Autodesk Inventor part; units mm, degrees
(part 2 of 3)
  arc A507 (33.3756, 32.7365) -> (33.2415, 32.8706) centre (33.2415, 32.7365) ccw
  arc A508 (33.3439, 32.7365) -> (33.4073, 32.7365) centre (33.3756, 32.7365) ccw
  arc A509 (33.2415, 32.9023) -> (33.2415, 32.8388) centre (33.2415, 32.8705) ccw
  line L202 (33.3756, 32.7365) -> (33.3756, 32.6025)
  arc A510 (33.3438, 32.6025) -> (33.4074, 32.6025) centre (33.3756, 32.6025) ccw
  arc A511 (33.4074, 32.7365) -> (33.3438, 32.7365) centre (33.3756, 32.7365) ccw
  arc A512 (33.0137, 33.4375) -> (32.893, 33.3169) centre (33.0137, 33.3168) ccw
  arc A513 (33.0137, 33.4058) -> (33.0137, 33.4693) centre (33.0137, 33.4376) ccw
  arc A514 (32.8612, 33.3169) -> (32.9247, 33.3169) centre (32.8929, 33.3169) ccw
  arc A515 (32.893, 33.3169) -> (33.0002, 33.1694) centre (33.048, 33.3168) ccw
  arc A516 (32.9247, 33.3169) -> (32.8613, 33.3169) centre (32.893, 33.3169) ccw
  arc A517 (32.9905, 33.1392) -> (33.01, 33.1996) centre (33.0002, 33.1694) ccw
  arc A518 (33.1075, 33.3973) -> (33.0137, 33.4375) centre (33.0137, 33.308) ccw
  arc A519 (33.0137, 33.4693) -> (33.0137, 33.4058) centre (33.0137, 33.4376) ccw
  line L203 (33.1075, 33.3973) -> (33.3756, 33.1694)
  arc A520 (33.355, 33.1452) -> (33.3962, 33.1936) centre (33.3756, 33.1694) ccw
  arc A521 (33.1281, 33.4215) -> (33.0869, 33.3731) centre (33.1075, 33.3973) ccw
  line L204 (33.3756, 33.1694) -> (33.3756, 33.4375)
  arc A522 (33.4074, 33.4375) -> (33.3438, 33.4375) centre (33.3756, 33.4375) ccw
  arc A523 (33.3438, 33.1694) -> (33.4074, 33.1694) centre (33.3756, 33.1694) ccw
  arc A524 (27.3812, 21.5392) -> (27.3304, 21.5392) centre (27.3558, 21.5392) ccw
  arc A525 (27.3304, 20.6502) -> (27.3812, 20.6502) centre (27.3558, 20.6502) ccw
  line L205 (27.3558, 21.5392) -> (27.6027, 21.5392)
  arc A526 (27.6027, 21.5138) -> (27.6027, 21.5646) centre (27.6027, 21.5392) ccw
  arc A527 (27.3558, 21.5646) -> (27.3558, 21.5138) centre (27.3558, 21.5392) ccw
  arc A528 (27.6027, 21.0453) -> (27.6027, 21.5392) centre (27.6027, 21.2923) ccw
  arc A529 (27.6027, 21.0707) -> (27.6027, 21.0199) centre (27.6027, 21.0453) ccw
  arc A530 (27.6027, 21.5646) -> (27.6027, 21.5138) centre (27.6027, 21.5392) ccw
  line L206 (27.6027, 21.0453) -> (27.3558, 21.0453)
  arc A531 (27.6027, 21.0199) -> (27.6027, 21.0707) centre (27.6027, 21.0453) ccw
  line L207 (27.8497, 20.6502) -> (27.6521, 21.0453)
  arc A532 (27.6748, 21.0567) -> (27.6294, 21.034) centre (27.6521, 21.0453) ccw
  arc A533 (27.827, 20.6388) -> (27.8724, 20.6616) centre (27.8497, 20.6502) ccw
  arc A534 (28.7347, 21.317) -> (28.5124, 21.5392) centre (28.5124, 21.3169) ccw
  arc A535 (28.7093, 21.317) -> (28.7601, 21.317) centre (28.7347, 21.317) ccw
  arc A536 (28.5124, 21.5646) -> (28.5124, 21.5138) centre (28.5124, 21.5392) ccw
  arc A537 (33.0845, 33.3754) -> (33.1305, 33.4192) centre (33.1075, 33.3973) ccw
  line L208 (23.8252, 31.5903) -> (22.9362, 31.5903)
  arc A538 (22.9362, 31.6157) -> (22.9362, 31.5649) centre (22.9362, 31.5903) ccw
  arc A539 (23.8252, 31.5649) -> (23.8252, 31.6157) centre (23.8252, 31.5903) ccw
  line L209 (22.9362, 31.5903) -> (22.9362, 31.8373)
  arc A540 (22.9616, 31.8373) -> (22.9108, 31.8373) centre (22.9362, 31.8373) ccw
  arc A541 (22.9108, 31.5903) -> (22.9616, 31.5903) centre (22.9362, 31.5903) ccw
  arc A542 (23.4301, 31.8373) -> (22.9362, 31.8373) centre (23.1831, 31.8373) ccw
  arc A543 (23.4047, 31.8373) -> (23.4555, 31.8373) centre (23.4301, 31.8373) ccw
  arc A544 (22.9108, 31.8373) -> (22.9616, 31.8373) centre (22.9362, 31.8373) ccw
  line L210 (23.4301, 31.8373) -> (23.4301, 31.5903)
  arc A545 (23.4047, 31.5903) -> (23.4555, 31.5903) centre (23.4301, 31.5903) ccw
  arc A546 (23.4555, 31.8373) -> (23.4047, 31.8373) centre (23.4301, 31.8373) ccw
  line L211 (23.8252, 32.0842) -> (23.4301, 31.8867)
  arc A547 (23.4187, 31.9094) -> (23.4414, 31.8639) centre (23.4301, 31.8867) ccw
  arc A548 (23.8366, 32.0615) -> (23.8138, 32.1069) centre (23.8252, 32.0842) ccw
  line L212 (22.9362, 32.6729) -> (23.6276, 32.4753)
  arc A549 (23.6207, 32.4509) -> (23.6346, 32.4997) centre (23.6276, 32.4753) ccw
  arc A550 (28.5124, 21.5392) -> (28.2408, 21.3416) centre (28.5124, 21.2537) ccw
  arc A551 (22.9432, 32.6973) -> (22.9292, 32.6484) centre (22.9362, 32.6728) ccw
  line L213 (23.6276, 32.4753) -> (23.6276, 32.9692)
  arc A552 (23.653, 32.9692) -> (23.6022, 32.9692) centre (23.6276, 32.9692) ccw
  arc A553 (23.6022, 32.4753) -> (23.653, 32.4753) centre (23.6276, 32.4753) ccw
  line L214 (23.4301, 32.821) -> (23.8252, 32.821)
  arc A554 (23.8252, 32.7956) -> (23.8252, 32.8464) centre (23.8252, 32.821) ccw
  arc A555 (23.4301, 32.8464) -> (23.4301, 32.7956) centre (23.4301, 32.821) ccw
  arc A556 (29.2213, 23.5458) -> (29.2721, 23.5458) centre (29.2467, 23.5458) ccw
  arc A557 (29.2721, 23.7927) -> (29.2213, 23.7927) centre (29.2467, 23.7927) ccw
  line L215 (29.6418, 24.0397) -> (29.2467, 23.8421)
  arc A558 (29.2353, 23.8648) -> (29.258, 23.8194) centre (29.2467, 23.8421) ccw
  arc A559 (29.6532, 24.017) -> (29.6304, 24.0624) centre (29.6418, 24.0397) ccw
  line L216 (29.6418, 24.4308) -> (29.6418, 24.6777)
  arc A560 (29.6672, 24.6777) -> (29.6164, 24.6777) centre (29.6418, 24.6777) ccw
  arc A561 (29.6164, 24.4308) -> (29.6672, 24.4308) centre (29.6418, 24.4308) ccw
  arc A562 (29.6418, 24.6777) -> (29.1479, 24.6777) centre (29.3948, 24.6777) ccw
  arc A563 (29.6164, 24.6777) -> (29.6672, 24.6777) centre (29.6418, 24.6777) ccw
  arc A564 (29.1225, 24.6777) -> (29.1733, 24.6777) centre (29.1479, 24.6777) ccw
  line L217 (28.7528, 24.4308) -> (28.7528, 24.7271)
  arc A565 (28.7782, 24.7271) -> (28.7274, 24.7271) centre (28.7528, 24.7271) ccw
  arc A566 (28.7274, 24.4308) -> (28.7782, 24.4308) centre (28.7528, 24.4308) ccw
  arc A567 (29.1479, 24.7271) -> (28.7528, 24.7271) centre (28.9504, 24.7271) ccw
  arc A568 (29.1225, 24.7271) -> (29.1733, 24.7271) centre (29.1479, 24.7271) ccw
  arc A569 (28.7274, 24.7271) -> (28.7782, 24.7271) centre (28.7528, 24.7271) ccw
  line L218 (29.1479, 24.7271) -> (29.1479, 24.5296)
  arc A570 (29.1225, 24.5296) -> (29.1733, 24.5296) centre (29.1479, 24.5296) ccw
  arc A571 (29.1733, 24.7271) -> (29.1225, 24.7271) centre (29.1479, 24.7271) ccw
  arc A572 (31.2023, 14.7715) -> (31.2023, 14.8223) centre (31.2023, 14.7969) ccw
  arc A573 (28.5124, 21.5138) -> (28.5124, 21.5646) centre (28.5124, 21.5392) ccw
  arc A574 (28.2166, 21.3495) -> (28.2649, 21.3338) centre (28.2408, 21.3417) ccw
  line L219 (31.4492, 14.4018) -> (31.2517, 14.7969)
  arc A575 (28.6606, 21.1441) -> (28.7347, 21.317) centre (28.496, 21.317) ccw
  arc A576 (28.6431, 21.1625) -> (28.6781, 21.1257) centre (28.6606, 21.1441) ccw
  arc A577 (28.7601, 21.3169) -> (28.7093, 21.317) centre (28.7347, 21.317) ccw
  line L220 (28.6606, 21.1441) -> (28.2408, 20.6502)
  line L221 (29.6418, 23.5458) -> (28.7528, 23.5458)
  arc A578 (28.7528, 23.5712) -> (28.7528, 23.5204) centre (28.7528, 23.5458) ccw
  arc A579 (29.6418, 23.5204) -> (29.6418, 23.5712) centre (29.6418, 23.5458) ccw
  line L222 (28.7528, 23.5458) -> (28.7528, 23.7927)
  arc A580 (28.7782, 23.7927) -> (28.7274, 23.7927) centre (28.7528, 23.7927) ccw
  arc A581 (28.7274, 23.5458) -> (28.7782, 23.5458) centre (28.7528, 23.5458) ccw
  arc A582 (29.2467, 23.7927) -> (28.7528, 23.7927) centre (28.9997, 23.7927) ccw
  arc A583 (29.2213, 23.7927) -> (29.2721, 23.7927) centre (29.2467, 23.7927) ccw
  arc A584 (28.2214, 20.6667) -> (28.2601, 20.6337) centre (28.2408, 20.6502) ccw
  arc A585 (28.6799, 21.1276) -> (28.6412, 21.1605) centre (28.6606, 21.1441) ccw
  line L223 (28.2408, 20.6502) -> (28.7347, 20.6502)
  arc A586 (28.7347, 20.6248) -> (28.7347, 20.6756) centre (28.7347, 20.6502) ccw
  arc A587 (28.2408, 20.6756) -> (28.2408, 20.6248) centre (28.2408, 20.6502) ccw
  arc A588 (31.2744, 14.8083) -> (31.2289, 14.7856) centre (31.2516, 14.7969) ccw
  arc A589 (30.9553, 14.8223) -> (30.9553, 14.7715) centre (30.9553, 14.7969) ccw
  line L224 (31.2023, 14.7969) -> (30.9553, 14.7969)
  arc A590 (31.2023, 15.3162) -> (31.2023, 15.2654) centre (31.2023, 15.2908) ccw
  arc A591 (31.2023, 14.8223) -> (31.2023, 14.7715) centre (31.2023, 14.7969) ccw
  arc A592 (31.2023, 14.7969) -> (31.2023, 15.2908) centre (31.2023, 15.0439) ccw
  arc A593 (30.9553, 15.3162) -> (30.9553, 15.2654) centre (30.9553, 15.2908) ccw
  arc A594 (31.2023, 15.2654) -> (31.2023, 15.3162) centre (31.2023, 15.2908) ccw
  line L225 (30.9553, 15.2908) -> (31.2023, 15.2908)
  arc A595 (30.9299, 14.4018) -> (30.9807, 14.4018) centre (30.9553, 14.4018) ccw
  arc A596 (30.9807, 15.2908) -> (30.9299, 15.2908) centre (30.9553, 15.2908) ccw
  line L226 (30.9553, 14.4018) -> (30.9553, 15.2908)
  arc A597 (31.4265, 14.3904) -> (31.4719, 14.4132) centre (31.4492, 14.4018) ccw
  arc A598 (41.6076, 4.6462) -> (41.6076, 4.5954) centre (41.6076, 4.6208) ccw
  arc A599 (42.2567, 4.5954) -> (42.2567, 4.6462) centre (42.2567, 4.6208) ccw
  line L227 (41.6076, 4.6208) -> (42.2567, 4.6208)
  arc A600 (42.1787, 5.2535) -> (42.14, 5.2864) centre (42.1594, 5.2699) ccw
  arc A601 (41.5883, 4.6373) -> (41.627, 4.6043) centre (41.6077, 4.6208) ccw
  line L228 (42.1594, 5.2699) -> (41.6076, 4.6208)
  arc A602 (42.2821, 5.4971) -> (42.2313, 5.4971) centre (42.2567, 5.4971) ccw
  arc A603 (42.1418, 5.2883) -> (42.1769, 5.2515) centre (42.1594, 5.2699) ccw
  arc A604 (42.1594, 5.2699) -> (42.2567, 5.4971) centre (41.943, 5.497) ccw
  arc A605 (41.5834, 5.5374) -> (41.6318, 5.5217) centre (41.6076, 5.5296) ccw
  arc A606 (41.9646, 5.7638) -> (41.9646, 5.8146) centre (41.9646, 5.7892) ccw
  arc A607 (41.9646, 5.7892) -> (41.6076, 5.5296) centre (41.9646, 5.414) ccw
  arc A608 (41.9646, 5.8146) -> (41.9646, 5.7638) centre (41.9646, 5.7892) ccw
  arc A609 (42.2313, 5.4971) -> (42.2821, 5.4971) centre (42.2567, 5.4971) ccw
  arc A610 (42.2567, 5.4971) -> (41.9646, 5.7892) centre (41.9646, 5.4971) ccw
  arc A611 (40.8206, 4.5954) -> (40.8206, 4.6462) centre (40.8206, 4.6208) ccw
  arc A612 (40.6908, 4.6462) -> (40.6908, 4.5954) centre (40.6908, 4.6208) ccw
  line L229 (40.8206, 4.6208) -> (40.6908, 4.6208)
  arc A613 (41.1057, 4.8804) -> (41.0549, 4.8804) centre (41.0803, 4.8804) ccw
  arc A614 (40.8206, 4.6462) -> (40.8206, 4.5954) centre (40.8206, 4.6208) ccw
  arc A615 (40.8206, 4.6208) -> (41.0803, 4.8804) centre (40.8206, 4.8805) ccw
  arc A616 (41.1057, 5.7892) -> (41.0549, 5.7892) centre (41.0803, 5.7892) ccw
  arc A617 (41.0549, 4.8804) -> (41.1057, 4.8804) centre (41.0803, 4.8804) ccw
  line L230 (41.0803, 5.7892) -> (41.0803, 4.8804)
  arc A618 (28.2702, 18.8976) -> (28.2702, 18.8468) centre (28.2702, 18.8722) ccw
  arc A619 (28.7641, 18.8468) -> (28.7641, 18.8976) centre (28.7641, 18.8722) ccw
  line L231 (28.2702, 18.8722) -> (28.7641, 18.8722)
  arc A620 (28.5425, 19.7612) -> (28.4917, 19.7612) centre (28.5171, 19.7612) ccw
  arc A621 (28.4917, 18.8722) -> (28.5425, 18.8722) centre (28.5171, 18.8722) ccw
  line L232 (28.5171, 19.7612) -> (28.5171, 18.8722)
  arc A622 (28.2543, 19.5835) -> (28.2861, 19.5438) centre (28.2702, 19.5637) ccw
  arc A623 (28.533, 19.7414) -> (28.5013, 19.781) centre (28.5172, 19.7612) ccw
  line L233 (28.2702, 19.5636) -> (28.5171, 19.7612)
  arc A624 (29.5815, 18.9957) -> (29.6556, 19.3167) centre (28.9231, 19.3167) ccw
  arc A625 (31.3975, 16.1676) -> (31.4421, 16.192) centre (31.4198, 16.1798) ccw
  arc A626 (31.1458, 16.7352) -> (31.1012, 16.7109) centre (31.1235, 16.7231) ccw
  line L234 (31.4198, 16.1798) -> (31.1235, 16.7231)
  arc A627 (31.4386, 17.0517) -> (31.401, 17.0859) centre (31.4198, 17.0688) ccw
  arc A628 (30.9071, 16.5426) -> (30.9447, 16.5084) centre (30.9259, 16.5255) ccw
  line L235 (31.4198, 17.0688) -> (30.9259, 16.5255)
  arc A629 (30.9005, 16.1798) -> (30.9513, 16.1798) centre (30.9259, 16.1798) ccw
  arc A630 (30.9513, 17.0688) -> (30.9005, 17.0688) centre (30.9259, 17.0688) ccw
  line L236 (30.9259, 16.1798) -> (30.9259, 17.0688)
  arc A631 (30.0191, 16.3932) -> (30.0588, 16.3615) centre (30.0389, 16.3773) ccw
  arc A632 (30.4539, 16.8554) -> (30.4143, 16.8871) centre (30.4341, 16.8712) ccw
  line L237 (30.039, 16.3774) -> (30.4341, 16.8712)
  arc A633 (30.4334, 16.295) -> (30.3854, 16.3115) centre (30.4094, 16.3032) ccw
  arc A634 (30.2365, 16.2052) -> (30.2365, 16.1544) centre (30.2365, 16.1798) ccw
  arc A635 (30.2365, 16.1798) -> (30.4094, 16.3033) centre (30.2365, 16.3626) ccw
  arc A636 (30.5089, 16.6243) -> (30.4581, 16.6243) centre (30.4835, 16.6243) ccw
  arc A637 (30.3866, 16.3144) -> (30.4322, 16.2921) centre (30.4094, 16.3032) ccw
  arc A638 (30.4094, 16.3033) -> (30.4835, 16.6243) centre (29.751, 16.6243) ccw
  arc A639 (30.2365, 16.1544) -> (30.2365, 16.2052) centre (30.2365, 16.1798) ccw
  arc A640 (30.0877, 16.3115) -> (30.0396, 16.295) centre (30.0637, 16.3032) ccw
  arc A641 (30.0637, 16.3033) -> (30.2365, 16.1798) centre (30.2365, 16.3625) ccw
  arc A642 (30.0408, 16.2921) -> (30.0865, 16.3144) centre (30.0637, 16.3032) ccw
  arc A643 (30.015, 16.6243) -> (29.9642, 16.6243) centre (29.9896, 16.6243) ccw
  arc A644 (29.9896, 16.6243) -> (30.0637, 16.3033) centre (30.7221, 16.6243) ccw
  arc A645 (30.4322, 16.9565) -> (30.3866, 16.9342) centre (30.4094, 16.9453) ccw
  arc A646 (30.4581, 16.6243) -> (30.5089, 16.6243) centre (30.4835, 16.6243) ccw
  arc A647 (30.4835, 16.6243) -> (30.4094, 16.9453) centre (29.751, 16.6243) ccw
  arc A648 (30.2365, 17.0942) -> (30.2365, 17.0434) centre (30.2365, 17.0688) ccw
  arc A649 (30.3854, 16.9371) -> (30.4334, 16.9536) centre (30.4094, 16.9454) ccw
  arc A650 (30.0396, 16.9536) -> (30.0877, 16.9371) centre (30.0637, 16.9454) ccw
  arc A651 (30.2365, 17.0434) -> (30.2365, 17.0942) centre (30.2365, 17.0688) ccw
  arc A652 (30.2365, 17.0688) -> (30.0637, 16.9453) centre (30.2365, 16.8861) ccw
  arc A653 (29.9642, 16.6243) -> (30.015, 16.6243) centre (29.9896, 16.6243) ccw
  arc A654 (30.0865, 16.9342) -> (30.0408, 16.9565) centre (30.0637, 16.9453) ccw
  arc A655 (30.0637, 16.9453) -> (29.9896, 16.6243) centre (30.7221, 16.6243) ccw
  arc A656 (29.0981, 16.2052) -> (29.0981, 16.1544) centre (29.0981, 16.1798) ccw
  arc A657 (29.5919, 16.1544) -> (29.5919, 16.2052) centre (29.5919, 16.1798) ccw
  line L238 (29.0981, 16.1798) -> (29.5919, 16.1798)
  arc A658 (29.3704, 17.0688) -> (29.3196, 17.0688) centre (29.345, 17.0688) ccw
  arc A659 (29.3196, 16.1798) -> (29.3704, 16.1798) centre (29.345, 16.1798) ccw
  line L239 (29.345, 17.0688) -> (29.345, 16.1798)
  arc A660 (29.0822, 16.8911) -> (29.1139, 16.8514) centre (29.0981, 16.8713) ccw
  arc A661 (29.3609, 17.049) -> (29.3291, 17.0886) centre (29.345, 17.0688) ccw
  line L240 (29.0981, 16.8712) -> (29.345, 17.0688)
  arc A662 (30.5697, 18.86) -> (30.6142, 18.8844) centre (30.592, 18.8722) ccw
  arc A663 (30.3179, 19.4276) -> (30.2733, 19.4033) centre (30.2956, 19.4154) ccw
  line L241 (30.592, 18.8722) -> (30.2956, 19.4155)
  arc A664 (30.6107, 19.7441) -> (30.5732, 19.7783) centre (30.592, 19.7612) ccw
  arc A665 (30.0793, 19.235) -> (30.1169, 19.2008) centre (30.0981, 19.2179) ccw
  line L242 (30.592, 19.7612) -> (30.0981, 19.2179)
  arc A666 (30.0727, 18.8722) -> (30.1235, 18.8722) centre (30.0981, 18.8722) ccw
  arc A667 (30.1235, 19.7612) -> (30.0727, 19.7612) centre (30.0981, 19.7612) ccw
  line L243 (30.0981, 18.8722) -> (30.0981, 19.7612)
  arc A668 (29.1913, 19.0856) -> (29.231, 19.0539) centre (29.2112, 19.0697) ccw
  arc A669 (29.6261, 19.5478) -> (29.5864, 19.5795) centre (29.6063, 19.5636) ccw
  line L244 (29.2111, 19.0698) -> (29.6062, 19.5636)
  arc A670 (29.6056, 18.9874) -> (29.5575, 19.0039) centre (29.5816, 18.9957) ccw
  arc A671 (29.4087, 18.8976) -> (29.4087, 18.8468) centre (29.4087, 18.8722) ccw
  arc A672 (29.4087, 18.8722) -> (29.5815, 18.9957) centre (29.4087, 19.0549) ccw
  arc A673 (29.681, 19.3167) -> (29.6302, 19.3167) centre (29.6556, 19.3167) ccw
  arc A674 (29.5587, 19.0068) -> (29.6044, 18.9845) centre (29.5816, 18.9956) ccw
  arc A675 (30.4094, 16.9453) -> (30.2365, 17.0688) centre (30.2365, 16.886) ccw
  arc A676 (29.4087, 18.8468) -> (29.4087, 18.8976) centre (29.4087, 18.8722) ccw
  arc A677 (29.2598, 19.0039) -> (29.2118, 18.9874) centre (29.2358, 18.9957) ccw
  arc A678 (29.2358, 18.9957) -> (29.4087, 18.8722) centre (29.4087, 19.055) ccw
  arc A679 (29.213, 18.9845) -> (29.2587, 19.0068) centre (29.2358, 18.9956) ccw
  arc A680 (29.1871, 19.3167) -> (29.1363, 19.3167) centre (29.1617, 19.3167) ccw
  arc A681 (29.1617, 19.3167) -> (29.2358, 18.9957) centre (29.8942, 19.3167) ccw
  arc A682 (29.6044, 19.6489) -> (29.5587, 19.6266) centre (29.5816, 19.6378) ccw
  arc A683 (29.6302, 19.3167) -> (29.681, 19.3167) centre (29.6556, 19.3167) ccw
  arc A684 (29.6556, 19.3167) -> (29.5815, 19.6377) centre (28.9231, 19.3167) ccw
  arc A685 (29.4087, 19.7866) -> (29.4087, 19.7358) centre (29.4087, 19.7612) ccw
  arc A686 (29.5575, 19.6295) -> (29.6056, 19.646) centre (29.5816, 19.6378) ccw
  arc A687 (29.5815, 19.6377) -> (29.4087, 19.7612) centre (29.4087, 19.5785) ccw
  arc A688 (29.2118, 19.646) -> (29.2598, 19.6295) centre (29.2358, 19.6378) ccw
  arc A689 (29.4087, 19.7358) -> (29.4087, 19.7866) centre (29.4087, 19.7612) ccw
  arc A690 (29.4087, 19.7612) -> (29.2358, 19.6377) centre (29.4087, 19.5784) ccw
  arc A691 (29.1363, 19.3167) -> (29.1871, 19.3167) centre (29.1617, 19.3167) ccw
  arc A692 (29.2587, 19.6266) -> (29.213, 19.6489) centre (29.2358, 19.6378) ccw
  arc A693 (29.2358, 19.6377) -> (29.1617, 19.3167) centre (29.8942, 19.3167) ccw
  arc A694 (21.463, 33.401) -> (21.717, 33.401) centre (21.59, 33.401) ccw
  line L245 (21.59, 34.29) -> (21.59, 33.401)
  arc A695 (34.671, 33.02) -> (36.83, 30.861) centre (36.83, 33.02) ccw
  arc A696 (35.179, 33.02) -> (36.83, 31.369) centre (36.83, 33.02) ccw
  arc A697 (37.973, 33.02) -> (36.83, 34.163) centre (36.83, 33.02) ccw
  arc A698 (35.687, 33.02) -> (36.83, 31.877) centre (36.83, 33.02) ccw
  arc A699 (24.765, 30.5308) -> (24.765, 30.4292) centre (24.765, 30.48) ccw
  arc A700 (28.575, 30.4292) -> (28.575, 30.5308) centre (28.575, 30.48) ccw
  line L246 (24.765, 30.48) -> (28.575, 30.48)
  arc A701 (24.511, 33.02) -> (26.67, 30.861) centre (26.67, 33.02) ccw
  arc A702 (28.829, 33.02) -> (26.67, 35.179) centre (26.67, 33.02) ccw
  arc A703 (25.019, 33.02) -> (26.67, 31.369) centre (26.67, 33.02) ccw
  arc A704 (28.321, 33.02) -> (26.67, 34.671) centre (26.67, 33.02) ccw
  arc A705 (25.527, 33.02) -> (26.67, 31.877) centre (26.67, 33.02) ccw
  arc A706 (27.813, 33.02) -> (26.67, 34.163) centre (26.67, 33.02) ccw
  arc A707 (21.463, 26.67) -> (21.717, 26.67) centre (21.59, 26.67) ccw
  arc A708 (21.717, 27.559) -> (21.463, 27.559) centre (21.59, 27.559) ccw
  line L247 (21.59, 26.67) -> (21.59, 27.559)
  arc A709 (30.861, 22.225) -> (31.115, 22.225) centre (30.988, 22.225) ccw
  line L248 (32.7604, 10.8692) -> (32.7604, 9.7008)
  arc A710 (32.4199, 10.6294) -> (32.4517, 10.5897) centre (32.4358, 10.6096) ccw
  arc A711 (32.7762, 10.8494) -> (32.7445, 10.889) centre (32.7604, 10.8692) ccw
  line L249 (32.4358, 10.6096) -> (32.7604, 10.8692)
  arc A712 (24.3483, -0.92) -> (24.4118, -0.92) centre (24.3801, -0.92) ccw
  arc A713 (24.4118, 12.08) -> (24.3483, 12.08) centre (24.3801, 12.08) ccw
  line L250 (24.38, -0.92) -> (24.38, 12.08)
  arc A714 (33.655, 16.51) -> (33.655, 16.764) centre (33.655, 16.637) ccw
  arc A715 (32.766, 16.764) -> (32.766, 16.51) centre (32.766, 16.637) ccw
  line L251 (33.655, 16.637) -> (32.766, 16.637)
  arc A716 (26.035, 16.764) -> (26.035, 16.51) centre (26.035, 16.637) ccw
  arc A717 (26.924, 16.51) -> (26.924, 16.764) centre (26.924, 16.637) ccw
  line L252 (26.035, 16.637) -> (26.924, 16.637)
  line L253 (30.988, 29.845) -> (30.988, 28.956)
  arc A718 (38.481, 33.02) -> (36.83, 34.671) centre (36.83, 33.02) ccw
  arc A719 (27.8751, 8.1788) -> (27.8751, 8.2296) centre (27.8751, 8.2042) ccw
  arc A720 (27.8751, 8.2042) -> (27.3558, 7.6849) centre (27.8751, 7.6849) ccw
  arc A721 (27.3304, 7.3604) -> (27.3812, 7.3604) centre (27.3558, 7.3604) ccw
  arc A722 (27.3812, 7.6849) -> (27.3304, 7.6849) centre (27.3558, 7.6849) ccw
  line L254 (27.3558, 7.3604) -> (27.3558, 7.6849)
  arc A723 (28.0303, 7.3604) -> (27.9795, 7.3604) centre (28.0049, 7.3604) ccw
  arc A724 (27.3812, 7.3604) -> (27.3304, 7.3604) centre (27.3558, 7.3604) ccw
  arc A725 (27.3558, 7.3604) -> (28.0049, 7.3604) centre (27.6803, 7.3604) ccw
  arc A726 (28.0303, 7.4253) -> (27.9795, 7.4253) centre (28.0049, 7.4253) ccw
  arc A727 (27.9795, 7.3604) -> (28.0303, 7.3604) centre (28.0049, 7.3604) ccw
  line L255 (28.0049, 7.4253) -> (28.0049, 7.3604)
  arc A728 (27.7453, 7.7103) -> (27.7453, 7.6595) centre (27.7453, 7.6849) ccw
  arc A729 (27.9795, 7.4253) -> (28.0303, 7.4253) centre (28.0049, 7.4253) ccw
  arc A730 (28.0049, 7.4253) -> (27.7453, 7.6849) centre (27.7453, 7.4253) ccw
  arc A731 (27.3558, 7.7103) -> (27.3558, 7.6595) centre (27.3558, 7.6849) ccw
  arc A732 (27.7453, 7.6595) -> (27.7453, 7.7103) centre (27.7453, 7.6849) ccw
  line L256 (27.3558, 7.6849) -> (27.7453, 7.6849)
  arc A733 (36.58, -0.9518) -> (36.58, -0.8882) centre (36.58, -0.92) ccw
  arc A734 (24.38, -0.8882) -> (24.38, -0.9518) centre (24.38, -0.92) ccw
  line L257 (36.58, -0.92) -> (24.38, -0.92)
  arc A735 (36.6118, 12.08) -> (36.5482, 12.08) centre (36.58, 12.08) ccw
  arc A736 (36.5482, -0.92) -> (36.6118, -0.92) centre (36.58, -0.92) ccw
  line L258 (36.58, 12.08) -> (36.58, -0.92)
  arc A737 (24.38, 12.1118) -> (24.38, 12.0482) centre (24.38, 12.08) ccw
  arc A738 (36.58, 12.0482) -> (36.58, 12.1118) centre (36.58, 12.08) ccw
  line L259 (24.38, 12.08) -> (36.58, 12.08)
  arc A739 (38.735, 35.5092) -> (38.735, 35.6108) centre (38.735, 35.56) ccw
  arc A740 (38.989, 33.02) -> (36.83, 35.179) centre (36.83, 33.02) ccw
  arc A741 (26.035, 19.431) -> (26.035, 19.177) centre (26.035, 19.304) ccw
  arc A742 (26.924, 19.177) -> (26.924, 19.431) centre (26.924, 19.304) ccw
  line L260 (26.035, 19.304) -> (26.924, 19.304)
  arc A743 (34.925, 35.6108) -> (34.925, 35.5092) centre (34.925, 35.56) ccw
  arc A744 (33.655, 19.177) -> (33.655, 19.431) centre (33.655, 19.304) ccw
  arc A745 (32.766, 19.431) -> (32.766, 19.177) centre (32.766, 19.304) ccw
  line L261 (33.655, 19.304) -> (32.766, 19.304)
  line L262 (38.735, 35.56) -> (34.925, 35.56)
  arc A746 (30.861, 28.956) -> (31.115, 28.956) centre (30.988, 28.956) ccw
  arc A747 (31.115, 29.845) -> (30.861, 29.845) centre (30.988, 29.845) ccw
  line L263 (30.988, 22.225) -> (30.988, 23.114)
  arc A748 (31.115, 23.114) -> (30.861, 23.114) centre (30.988, 23.114) ccw
  arc A749 (21.717, 34.29) -> (21.463, 34.29) centre (21.59, 34.29) ccw
  arc A750 (32.4358, 9.7262) -> (32.4358, 9.6754) centre (32.4358, 9.7008) ccw
  arc A751 (33.0849, 9.6754) -> (33.0849, 9.7262) centre (33.0849, 9.7008) ccw
  line L264 (32.4358, 9.7008) -> (33.0849, 9.7008)
  arc A752 (32.7858, 10.8692) -> (32.735, 10.8692) centre (32.7604, 10.8692) ccw
  arc A753 (32.735, 9.7008) -> (32.7858, 9.7008) centre (32.7604, 9.7008) ccw
  arc A754 (27.3304, 7.6849) -> (27.3812, 7.6849) centre (27.3558, 7.6849) ccw
  arc A755 (26.2001, 34.29) -> (27.1399, 34.29) centre (26.67, 34.29) ccw
  arc A756 (27.1399, 34.29) -> (26.2001, 34.29) centre (26.67, 34.29) ccw
  arc A757 (26.2001, 34.29) -> (27.1399, 34.29) centre (26.67, 34.29) ccw
  arc A758 (27.1399, 34.29) -> (26.2001, 34.29) centre (26.67, 34.29) ccw
  arc A759 (26.2001, 31.75) -> (27.1399, 31.75) centre (26.67, 31.75) ccw
  arc A760 (27.1399, 31.75) -> (26.2001, 31.75) centre (26.67, 31.75) ccw
  arc A761 (26.2001, 31.75) -> (27.1399, 31.75) centre (26.67, 31.75) ccw
  arc A762 (27.1399, 31.75) -> (26.2001, 31.75) centre (26.67, 31.75) ccw
  arc A763 (37.2999, 31.75) -> (36.3601, 31.75) centre (36.83, 31.75) ccw
  arc A764 (36.3601, 31.75) -> (37.2999, 31.75) centre (36.83, 31.75) ccw
  arc A765 (37.2999, 31.75) -> (36.3601, 31.75) centre (36.83, 31.75) ccw
  arc A766 (36.3601, 31.75) -> (37.2999, 31.75) centre (36.83, 31.75) ccw
  arc A767 (37.2999, 34.29) -> (36.3601, 34.29) centre (36.83, 34.29) ccw
  arc A768 (36.3601, 34.29) -> (37.2999, 34.29) centre (36.83, 34.29) ccw
  arc A769 (37.2999, 34.29) -> (36.3601, 34.29) centre (36.83, 34.29) ccw
  arc A770 (36.3601, 34.29) -> (37.2999, 34.29) centre (36.83, 34.29) ccw
  arc A771 (44.704, 11.942) -> (44.704, 12.696) centre (44.704, 12.319) ccw
  arc A772 (44.704, 12.696) -> (44.704, 11.942) centre (44.704, 12.319) ccw
  arc A773 (44.704, 11.942) -> (44.704, 12.696) centre (44.704, 12.319) ccw
  arc A774 (44.704, 12.696) -> (44.704, 11.942) centre (44.704, 12.319) ccw
  arc A775 (42.164, 11.942) -> (42.164, 12.696) centre (42.164, 12.319) ccw
  arc A776 (42.164, 12.696) -> (42.164, 11.942) centre (42.164, 12.319) ccw
  arc A777 (42.164, 11.942) -> (42.164, 12.696) centre (42.164, 12.319) ccw
  arc A778 (42.164, 12.696) -> (42.164, 11.942) centre (42.164, 12.319) ccw
  arc A779 (39.624, 11.942) -> (39.624, 12.696) centre (39.624, 12.319) ccw
  arc A780 (39.624, 12.696) -> (39.624, 11.942) centre (39.624, 12.319) ccw
  arc A781 (39.624, 11.942) -> (39.624, 12.696) centre (39.624, 12.319) ccw
  arc A782 (39.624, 12.696) -> (39.624, 11.942) centre (39.624, 12.319) ccw
  arc A783 (33.03, 9.568) -> (33.03, 10.272) centre (33.03, 9.92) ccw
  arc A784 (33.03, 10.272) -> (33.03, 9.568) centre (33.03, 9.92) ccw
  arc A785 (33.03, 9.568) -> (33.03, 10.272) centre (33.03, 9.92) ccw
  arc A786 (33.03, 10.272) -> (33.03, 9.568) centre (33.03, 9.92) ccw
  arc A787 (32.01, 7.028) -> (32.01, 7.732) centre (32.01, 7.38) ccw
  arc A788 (32.01, 7.732) -> (32.01, 7.028) centre (32.01, 7.38) ccw
  arc A789 (32.01, 7.028) -> (32.01, 7.732) centre (32.01, 7.38) ccw
  arc A790 (32.01, 7.732) -> (32.01, 7.028) centre (32.01, 7.38) ccw
  arc A791 (30.99, 9.568) -> (30.99, 10.272) centre (30.99, 9.92) ccw
  arc A792 (30.99, 10.272) -> (30.99, 9.568) centre (30.99, 9.92) ccw
  arc A793 (30.99, 9.568) -> (30.99, 10.272) centre (30.99, 9.92) ccw
  arc A794 (30.99, 10.272) -> (30.99, 9.568) centre (30.99, 9.92) ccw
  arc A795 (29.97, 7.028) -> (29.97, 7.732) centre (29.97, 7.38) ccw
  arc A796 (29.97, 7.732) -> (29.97, 7.028) centre (29.97, 7.38) ccw
  arc A797 (29.97, 7.028) -> (29.97, 7.732) centre (29.97, 7.38) ccw
  arc A798 (29.97, 7.732) -> (29.97, 7.028) centre (29.97, 7.38) ccw
  arc A799 (28.95, 9.568) -> (28.95, 10.272) centre (28.95, 9.92) ccw
  arc A800 (28.95, 10.272) -> (28.95, 9.568) centre (28.95, 9.92) ccw
  arc A801 (28.95, 9.568) -> (28.95, 10.272) centre (28.95, 9.92) ccw
  arc A802 (28.95, 10.272) -> (28.95, 9.568) centre (28.95, 9.92) ccw
  arc A803 (27.93, 7.028) -> (27.93, 7.732) centre (27.93, 7.38) ccw
  arc A804 (27.93, 7.732) -> (27.93, 7.028) centre (27.93, 7.38) ccw
  arc A805 (27.93, 7.028) -> (27.93, 7.732) centre (27.93, 7.38) ccw
  arc A806 (27.93, 7.732) -> (27.93, 7.028) centre (27.93, 7.38) ccw
  line L265 (27.6145, 17.137) -> (26.6145, 17.137)
  line L266 (26.6145, 17.137) -> (26.6145, 16.137)
  line L267 (26.6145, 16.137) -> (27.6145, 16.137)
  line L268 (27.6145, 16.137) -> (27.6145, 17.137)
  line L269 (33.0755, 17.137) -> (32.0755, 17.137)
  line L270 (32.0755, 17.137) -> (32.0755, 16.137)
  line L271 (32.0755, 16.137) -> (33.0755, 16.137)
  line L272 (33.0755, 16.137) -> (33.0755, 17.137)
  line L273 (34.1376, 16.837) -> (34.1376, 16.437)
  line L274 (34.1376, 16.437) -> (33.855, 16.1544)
  line L275 (33.855, 16.1544) -> (33.455, 16.1544)
  line L276 (33.455, 16.1544) -> (33.1724, 16.437)
  line L277 (33.1724, 16.437) -> (33.1724, 16.837)
  line L278 (33.1724, 16.837) -> (33.455, 17.1196)
  line L279 (33.455, 17.1196) -> (33.855, 17.1196)
  line L280 (33.855, 17.1196) -> (34.1376, 16.837)
  line L281 (34.1376, 16.837) -> (34.1376, 16.437)
  line L282 (34.1376, 16.837) -> (34.1376, 16.437)
  line L283 (34.1376, 16.437) -> (33.855, 16.1544)
  line L284 (33.855, 16.1544) -> (33.455, 16.1544)
  line L285 (33.455, 16.1544) -> (33.1724, 16.437)
  line L286 (33.1724, 16.437) -> (33.1724, 16.837)
  line L287 (33.1724, 16.837) -> (33.455, 17.1196)
  line L288 (33.455, 17.1196) -> (33.855, 17.1196)
  line L289 (33.855, 17.1196) -> (34.1376, 16.837)
  line L290 (34.1376, 16.837) -> (34.1376, 16.437)
  line L291 (26.5176, 16.837) -> (26.5176, 16.437)
  line L292 (26.5176, 16.437) -> (26.235, 16.1544)
  line L293 (26.235, 16.1544) -> (25.835, 16.1544)
  line L294 (25.835, 16.1544) -> (25.5524, 16.437)
  line L295 (25.5524, 16.437) -> (25.5524, 16.837)
  line L296 (25.5524, 16.837) -> (25.835, 17.1196)
  line L297 (25.835, 17.1196) -> (26.235, 17.1196)
  line L298 (26.235, 17.1196) -> (26.5176, 16.837)
  line L299 (26.5176, 16.837) -> (26.5176, 16.437)
  line L300 (26.5176, 16.837) -> (26.5176, 16.437)
  line L301 (26.5176, 16.437) -> (26.235, 16.1544)
  line L302 (26.235, 16.1544) -> (25.835, 16.1544)
  line L303 (25.835, 16.1544) -> (25.5524, 16.437)
  line L304 (25.5524, 16.437) -> (25.5524, 16.837)
  line L305 (25.5524, 16.837) -> (25.835, 17.1196)
  line L306 (25.835, 17.1196) -> (26.235, 17.1196)
  line L307 (26.235, 17.1196) -> (26.5176, 16.837)
  line L308 (26.5176, 16.837) -> (26.5176, 16.437)
  line L309 (32.0755, 18.804) -> (33.0755, 18.804)
  line L310 (33.0755, 18.804) -> (33.0755, 19.804)
  line L311 (33.0755, 19.804) -> (32.0755, 19.804)
  line L312 (32.0755, 19.804) -> (32.0755, 18.804)
  line L313 (26.6145, 18.804) -> (27.6145, 18.804)
  line L314 (27.6145, 18.804) -> (27.6145, 19.804)
  line L315 (27.6145, 19.804) -> (26.6145, 19.804)
  line L316 (26.6145, 19.804) -> (26.6145, 18.804)
  line L317 (25.5524, 19.104) -> (25.5524, 19.504)
  line L318 (25.5524, 19.504) -> (25.835, 19.7866)
  line L319 (25.835, 19.7866) -> (26.235, 19.7866)
  line L320 (26.235, 19.7866) -> (26.5176, 19.504)
  line L321 (26.5176, 19.504) -> (26.5176, 19.104)
  line L322 (26.5176, 19.104) -> (26.235, 18.8214)
  line L323 (26.235, 18.8214) -> (25.835, 18.8214)
  line L324 (25.835, 18.8214) -> (25.5524, 19.104)
  line L325 (25.5524, 19.104) -> (25.5524, 19.504)
  line L326 (25.5524, 19.104) -> (25.5524, 19.504)
  line L327 (25.5524, 19.504) -> (25.835, 19.7866)
  line L328 (25.835, 19.7866) -> (26.235, 19.7866)
  line L329 (26.235, 19.7866) -> (26.5176, 19.504)
  line L330 (26.5176, 19.504) -> (26.5176, 19.104)
  line L331 (26.5176, 19.104) -> (26.235, 18.8214)
  line L332 (26.235, 18.8214) -> (25.835, 18.8214)
  line L333 (25.835, 18.8214) -> (25.5524, 19.104)
  line L334 (25.5524, 19.104) -> (25.5524, 19.504)
  line L335 (33.1724, 19.104) -> (33.1724, 19.504)
  line L336 (33.1724, 19.504) -> (33.455, 19.7866)
  line L337 (33.455, 19.7866) -> (33.855, 19.7866)
  line L338 (33.855, 19.7866) -> (34.1376, 19.504)
  line L339 (34.1376, 19.504) -> (34.1376, 19.104)
  line L340 (34.1376, 19.104) -> (33.855, 18.8214)
  line L341 (33.855, 18.8214) -> (33.455, 18.8214)
  line L342 (33.455, 18.8214) -> (33.1724, 19.104)
  line L343 (33.1724, 19.104) -> (33.1724, 19.504)
  line L344 (33.1724, 19.104) -> (33.1724, 19.504)
  line L345 (33.1724, 19.504) -> (33.455, 19.7866)
  line L346 (33.455, 19.7866) -> (33.855, 19.7866)
  line L347 (33.855, 19.7866) -> (34.1376, 19.504)
  line L348 (34.1376, 19.504) -> (34.1376, 19.104)
  line L349 (34.1376, 19.104) -> (33.855, 18.8214)
  line L350 (33.855, 18.8214) -> (33.455, 18.8214)
  line L351 (33.455, 18.8214) -> (33.1724, 19.104)
  line L352 (33.1724, 19.104) -> (33.1724, 19.504)
  line L353 (31.488, 28.2655) -> (31.488, 29.2655)
  line L354 (31.488, 29.2655) -> (30.488, 29.2655)
  line L355 (30.488, 29.2655) -> (30.488, 28.2655)
  line L356 (30.488, 28.2655) -> (31.488, 28.2655)
  line L357 (31.488, 22.8045) -> (31.488, 23.8045)
  line L358 (31.488, 23.8045) -> (30.488, 23.8045)
  line L359 (30.488, 23.8045) -> (30.488, 22.8045)
  line L360 (30.488, 22.8045) -> (31.488, 22.8045)
  line L361 (31.188, 21.7424) -> (30.788, 21.7424)
  line L362 (30.788, 21.7424) -> (30.5054, 22.025)
  line L363 (30.5054, 22.025) -> (30.5054, 22.425)
  line L364 (30.5054, 22.425) -> (30.788, 22.7076)
  line L365 (30.788, 22.7076) -> (31.188, 22.7076)
  line L366 (31.188, 22.7076) -> (31.4706, 22.425)
  line L367 (31.4706, 22.425) -> (31.4706, 22.025)
  line L368 (31.4706, 22.025) -> (31.188, 21.7424)
  line L369 (31.188, 21.7424) -> (30.788, 21.7424)
  line L370 (31.188, 21.7424) -> (30.788, 21.7424)
  line L371 (30.788, 21.7424) -> (30.5054, 22.025)
  line L372 (30.5054, 22.025) -> (30.5054, 22.425)
  line L373 (30.5054, 22.425) -> (30.788, 22.7076)
  line L374 (30.788, 22.7076) -> (31.188, 22.7076)
  line L375 (31.188, 22.7076) -> (31.4706, 22.425)
  line L376 (31.4706, 22.425) -> (31.4706, 22.025)
  line L377 (31.4706, 22.025) -> (31.188, 21.7424)
  line L378 (31.188, 21.7424) -> (30.788, 21.7424)
  line L379 (31.188, 29.3624) -> (30.788, 29.3624)
  line L380 (30.788, 29.3624) -> (30.5054, 29.645)
  line L381 (30.5054, 29.645) -> (30.5054, 30.045)
  line L382 (30.5054, 30.045) -> (30.788, 30.3276)
  line L383 (30.788, 30.3276) -> (31.188, 30.3276)
  line L384 (31.188, 30.3276) -> (31.4706, 30.045)
  line L385 (31.4706, 30.045) -> (31.4706, 29.645)
  line L386 (31.4706, 29.645) -> (31.188, 29.3624)
  line L387 (31.188, 29.3624) -> (30.788, 29.3624)
  line L388 (31.188, 29.3624) -> (30.788, 29.3624)
  line L389 (30.788, 29.3624) -> (30.5054, 29.645)
  line L390 (30.5054, 29.645) -> (30.5054, 30.045)
  line L391 (30.5054, 30.045) -> (30.788, 30.3276)
  line L392 (30.788, 30.3276) -> (31.188, 30.3276)
  line L393 (31.188, 30.3276) -> (31.4706, 30.045)
  line L394 (31.4706, 30.045) -> (31.4706, 29.645)
  line L395 (31.4706, 29.645) -> (31.188, 29.3624)
  line L396 (31.188, 29.3624) -> (30.788, 29.3624)
  line L397 (21.09, 28.2495) -> (21.09, 27.2495)
  line L398 (21.09, 27.2495) -> (22.09, 27.2495)
  line L399 (22.09, 27.2495) -> (22.09, 28.2495)
  line L400 (22.09, 28.2495) -> (21.09, 28.2495)
  line L401 (21.09, 33.7105) -> (21.09, 32.7105)
  line L402 (21.09, 32.7105) -> (22.09, 32.7105)
  line L403 (22.09, 32.7105) -> (22.09, 33.7105)
  line L404 (22.09, 33.7105) -> (21.09, 33.7105)
  line L405 (21.39, 34.7726) -> (21.79, 34.7726)
  line L406 (21.79, 34.7726) -> (22.0726, 34.49)
  line L407 (22.0726, 34.49) -> (22.0726, 34.09)
  line L408 (22.0726, 34.09) -> (21.79, 33.8074)
  line L409 (21.79, 33.8074) -> (21.39, 33.8074)
  line L410 (21.39, 33.8074) -> (21.1074, 34.09)
  line L411 (21.1074, 34.09) -> (21.1074, 34.49)
  line L412 (21.1074, 34.49) -> (21.39, 34.7726)
  line L413 (21.39, 34.7726) -> (21.79, 34.7726)
  line L414 (21.39, 34.7726) -> (21.79, 34.7726)
  line L415 (21.79, 34.7726) -> (22.0726, 34.49)
  line L416 (22.0726, 34.49) -> (22.0726, 34.09)
  line L417 (22.0726, 34.09) -> (21.79, 33.8074)
  line L418 (21.79, 33.8074) -> (21.39, 33.8074)
  line L419 (21.39, 33.8074) -> (21.1074, 34.09)
  line L420 (21.1074, 34.09) -> (21.1074, 34.49)
  line L421 (21.1074, 34.49) -> (21.39, 34.7726)
  line L422 (21.39, 34.7726) -> (21.79, 34.7726)
  line L423 (21.39, 27.1526) -> (21.79, 27.1526)
  line L424 (21.79, 27.1526) -> (22.0726, 26.87)
  line L425 (22.0726, 26.87) -> (22.0726, 26.47)
  line L426 (22.0726, 26.47) -> (21.79, 26.1874)
  line L427 (21.79, 26.1874) -> (21.39, 26.1874)
  line L428 (21.39, 26.1874) -> (21.1074, 26.47)
  line L429 (21.1074, 26.47) -> (21.1074, 26.87)
  line L430 (21.1074, 26.87) -> (21.39, 27.1526)
  line L431 (21.39, 27.1526) -> (21.79, 27.1526)
  line L432 (21.39, 27.1526) -> (21.79, 27.1526)
  line L433 (21.79, 27.1526) -> (22.0726, 26.87)
  line L434 (22.0726, 26.87) -> (22.0726, 26.47)
  line L435 (22.0726, 26.47) -> (21.79, 26.1874)
  line L436 (21.79, 26.1874) -> (21.39, 26.1874)
  line L437 (21.39, 26.1874) -> (21.1074, 26.47)
  line L438 (21.1074, 26.47) -> (21.1074, 26.87)
  line L439 (21.1074, 26.87) -> (21.39, 27.1526)
  line L440 (21.39, 27.1526) -> (21.79, 27.1526)
  arc A807 (37.773, 16.891) -> (38.427, 16.891) centre (38.1, 16.891) ccw
  arc A808 (38.427, 16.891) -> (37.773, 16.891) centre (38.1, 16.891) ccw
  arc A809 (37.773, 16.891) -> (38.427, 16.891) centre (38.1, 16.891) ccw
  arc A810 (38.427, 16.891) -> (37.773, 16.891) centre (38.1, 16.891) ccw
  arc A811 (37.773, 19.431) -> (38.427, 19.431) centre (38.1, 19.431) ccw
  arc A812 (38.427, 19.431) -> (37.773, 19.431) centre (38.1, 19.431) ccw
  arc A813 (37.773, 19.431) -> (38.427, 19.431) centre (38.1, 19.431) ccw
  arc A814 (38.427, 19.431) -> (37.773, 19.431) centre (38.1, 19.431) ccw
  arc A815 (37.773, 21.971) -> (38.427, 21.971) centre (38.1, 21.971) ccw
  arc A816 (38.427, 21.971) -> (37.773, 21.971) centre (38.1, 21.971) ccw
  arc A817 (37.773, 21.971) -> (38.427, 21.971) centre (38.1, 21.971) ccw
  arc A818 (38.427, 21.971) -> (37.773, 21.971) centre (38.1, 21.971) ccw
  arc A819 (37.773, 24.511) -> (38.427, 24.511) centre (38.1, 24.511) ccw
  arc A820 (38.427, 24.511) -> (37.773, 24.511) centre (38.1, 24.511) ccw
  arc A821 (37.773, 24.511) -> (38.427, 24.511) centre (38.1, 24.511) ccw
  arc A822 (38.427, 24.511) -> (37.773, 24.511) centre (38.1, 24.511) ccw
  arc A823 (22.5645, 17.018) -> (21.8855, 17.018) centre (22.225, 17.018) ccw
  arc A824 (21.8855, 17.018) -> (22.5645, 17.018) centre (22.225, 17.018) ccw
  arc A825 (22.5645, 17.018) -> (21.8855, 17.018) centre (22.225, 17.018) ccw
  arc A826 (21.8855, 17.018) -> (22.5645, 17.018) centre (22.225, 17.018) ccw
  arc A827 (22.5645, 22.098) -> (21.8855, 22.098) centre (22.225, 22.098) ccw
  arc A828 (21.8855, 22.098) -> (22.5645, 22.098) centre (22.225, 22.098) ccw
  arc A829 (22.5645, 22.098) -> (21.8855, 22.098) centre (22.225, 22.098) ccw
  arc A830 (21.8855, 22.098) -> (22.5645, 22.098) centre (22.225, 22.098) ccw
  arc A831 (22.5645, 19.558) -> (21.8855, 19.558) centre (22.225, 19.558) ccw
  arc A832 (21.8855, 19.558) -> (22.5645, 19.558) centre (22.225, 19.558) ccw
  arc A833 (22.5645, 19.558) -> (21.8855, 19.558) centre (22.225, 19.558) ccw
  arc A834 (21.8855, 19.558) -> (22.5645, 19.558) centre (22.225, 19.558) ccw
  arc A835 (27.051, 12.9975) -> (27.051, 13.6725) centre (27.051, 13.335) ccw
  arc A836 (27.051, 13.6725) -> (27.051, 12.9975) centre (27.051, 13.335) ccw
  arc A837 (27.051, 12.9975) -> (27.051, 13.6725) centre (27.051, 13.335) ccw
  arc A838 (27.051, 13.6725) -> (27.051, 12.9975) centre (27.051, 13.335) ccw
  arc A839 (30.988, 12.9975) -> (30.988, 13.6725) centre (30.988, 13.335) ccw
  arc A840 (30.988, 13.6725) -> (30.988, 12.9975) centre (30.988, 13.335) ccw
  arc A841 (30.988, 12.9975) -> (30.988, 13.6725) centre (30.988, 13.335) ccw
  arc A842 (30.988, 13.6725) -> (30.988, 12.9975) centre (30.988, 13.335) ccw
  arc A843 (33.655, 26.3325) -> (33.655, 27.0075) centre (33.655, 26.67) ccw
  arc A844 (33.655, 27.0075) -> (33.655, 26.3325) centre (33.655, 26.67) ccw
  arc A845 (33.655, 26.3325) -> (33.655, 27.0075) centre (33.655, 26.67) ccw
  arc A846 (33.655, 27.0075) -> (33.655, 26.3325) centre (33.655, 26.67) ccw
  arc A847 (33.655, 22.1415) -> (33.655, 22.8165) centre (33.655, 22.479) ccw
  arc A848 (33.655, 22.8165) -> (33.655, 22.1415) centre (33.655, 22.479) ccw
  arc A849 (33.655, 22.1415) -> (33.655, 22.8165) centre (33.655, 22.479) ccw
  arc A850 (33.655, 22.8165) -> (33.655, 22.1415) centre (33.655, 22.479) ccw
  line L441 (-13.871, -1.143) -> (46.533, -1.143)
  line L442 (46.533, -1.143) -> (46.533, 36.947)
  line L443 (46.533, 36.947) -> (-13.871, 36.947)
  line L444 (-13.871, 36.947) -> (-13.871, -1.143)
  point P0 (0, 0)
  point P1 (30.48, 5.08)
  point P2 (29.845, 19.304)
  point P3 (21.59, 30.48)
  point P4 (22.225, 24.638)
  point P5 (30.988, 26.035)
  point P6 (29.845, 16.637)
  constraints: 1686 point on circle, 890 end point, 851 centre point, 2 parallel, 1 horizontal, 1 perpendicular